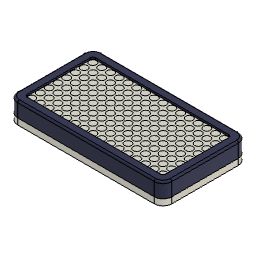
clock v5 (Autodesk Fusion 360 design; units mm, degrees)
Autodesk Fusion 360 part; units mm, degrees
(part 1 of 4)
sketch "Sketch1" plane through (0, 0, 0) normal (0, 0, 1) x (1, 0, 0)
  line L0 (1, 8.4943) -> (1, 1.4943)
  line L1 (1, 1.4943) -> (9, 1.4943)
  line L2 (9, 1.4943) -> (9, 8.4943)
  line L3 (9, 8.4943) -> (1, 8.4943)
  line L4 (19, 1.4943) -> (19, 8.4943)
  line L5 (19, 8.4943) -> (11, 8.4943)
  line L6 (11, 8.4943) -> (11, 1.4943)
  line L7 (11, 1.4943) -> (19, 1.4943)
  line L8 (29, 1.4943) -> (29, 8.4943)
  line L9 (29, 8.4943) -> (21, 8.4943)
  line L10 (21, 8.4943) -> (21, 1.4943)
  line L11 (21, 1.4943) -> (29, 1.4943)
  line L12 (39, 1.4943) -> (39, 8.4943)
  line L13 (39, 8.4943) -> (31, 8.4943)
  line L14 (31, 8.4943) -> (31, 1.4943)
  line L15 (31, 1.4943) -> (39, 1.4943)
  line L16 (49, 1.4943) -> (49, 8.4943)
  line L17 (49, 8.4943) -> (41, 8.4943)
  line L18 (41, 8.4943) -> (41, 1.4943)
  line L19 (41, 1.4943) -> (49, 1.4943)
  line L20 (59, 1.4943) -> (59, 8.4943)
  line L21 (59, 8.4943) -> (51, 8.4943)
  line L22 (51, 8.4943) -> (51, 1.4943)
  line L23 (51, 1.4943) -> (59, 1.4943)
  line L24 (69, 1.4943) -> (69, 8.4943)
  line L25 (69, 8.4943) -> (61, 8.4943)
  line L26 (61, 8.4943) -> (61, 1.4943)
  line L27 (61, 1.4943) -> (69, 1.4943)
  line L28 (79, 1.4943) -> (79, 8.4943)
  line L29 (79, 8.4943) -> (71, 8.4943)
  line L30 (71, 8.4943) -> (71, 1.4943)
  line L31 (71, 1.4943) -> (79, 1.4943)
  line L32 (89, 1.4943) -> (89, 8.4943)
  line L33 (89, 8.4943) -> (81, 8.4943)
  line L34 (81, 8.4943) -> (81, 1.4943)
  line L35 (81, 1.4943) -> (89, 1.4943)
  line L36 (99, 1.4943) -> (99, 8.4943)
  line L37 (99, 8.4943) -> (91, 8.4943)
  line L38 (91, 8.4943) -> (91, 1.4943)
  line L39 (91, 1.4943) -> (99, 1.4943)
  line L40 (109, 1.4943) -> (109, 8.4943)
  line L41 (109, 8.4943) -> (101, 8.4943)
  line L42 (101, 8.4943) -> (101, 1.4943)
  line L43 (101, 1.4943) -> (109, 1.4943)
  line L44 (119, 1.4943) -> (119, 8.4943)
  line L45 (119, 8.4943) -> (111, 8.4943)
  line L46 (111, 8.4943) -> (111, 1.4943)
  line L47 (111, 1.4943) -> (119, 1.4943)
  line L48 (129, 1.4943) -> (129, 8.4943)
  line L49 (129, 8.4943) -> (121, 8.4943)
  line L50 (121, 8.4943) -> (121, 1.4943)
  line L51 (121, 1.4943) -> (129, 1.4943)
  line L52 (139, 1.4943) -> (139, 8.4943)
  line L53 (139, 8.4943) -> (131, 8.4943)
  line L54 (131, 8.4943) -> (131, 1.4943)
  line L55 (131, 1.4943) -> (139, 1.4943)
  line L56 (149, 1.4943) -> (149, 8.4943)
  line L57 (149, 8.4943) -> (141, 8.4943)
  line L58 (141, 8.4943) -> (141, 1.4943)
  line L59 (141, 1.4943) -> (149, 1.4943)
  line L60 (159, 1.4943) -> (159, 8.4943)
  line L61 (159, 8.4943) -> (151, 8.4943)
  line L62 (151, 8.4943) -> (151, 1.4943)
  line L63 (151, 1.4943) -> (159, 1.4943)
  line L64 (9, 11.4943) -> (9, 18.4943)
  line L65 (9, 18.4943) -> (1, 18.4943)
  line L66 (1, 18.4943) -> (1, 11.4943)
  line L67 (1, 11.4943) -> (9, 11.4943)
  line L68 (19, 11.4943) -> (19, 18.4943)
  line L69 (19, 18.4943) -> (11, 18.4943)
  line L70 (11, 18.4943) -> (11, 11.4943)
  line L71 (11, 11.4943) -> (19, 11.4943)
  line L72 (29, 11.4943) -> (29, 18.4943)
  line L73 (29, 18.4943) -> (21, 18.4943)
  line L74 (21, 18.4943) -> (21, 11.4943)
  line L75 (21, 11.4943) -> (29, 11.4943)
  line L76 (39, 11.4943) -> (39, 18.4943)
  line L77 (39, 18.4943) -> (31, 18.4943)
  line L78 (31, 18.4943) -> (31, 11.4943)
  line L79 (31, 11.4943) -> (39, 11.4943)
  line L80 (49, 11.4943) -> (49, 18.4943)
  line L81 (49, 18.4943) -> (41, 18.4943)
  line L82 (41, 18.4943) -> (41, 11.4943)
  line L83 (41, 11.4943) -> (49, 11.4943)
  line L84 (59, 11.4943) -> (59, 18.4943)
  line L85 (59, 18.4943) -> (51, 18.4943)
  line L86 (51, 18.4943) -> (51, 11.4943)
  line L87 (51, 11.4943) -> (59, 11.4943)
  line L88 (69, 11.4943) -> (69, 18.4943)
  line L89 (69, 18.4943) -> (61, 18.4943)
  line L90 (61, 18.4943) -> (61, 11.4943)
  line L91 (61, 11.4943) -> (69, 11.4943)
  line L92 (79, 11.4943) -> (79, 18.4943)
  line L93 (79, 18.4943) -> (71, 18.4943)
  line L94 (71, 18.4943) -> (71, 11.4943)
  line L95 (71, 11.4943) -> (79, 11.4943)
  line L96 (89, 11.4943) -> (89, 18.4943)
  line L97 (89, 18.4943) -> (81, 18.4943)
  line L98 (81, 18.4943) -> (81, 11.4943)
  line L99 (81, 11.4943) -> (89, 11.4943)
  line L100 (99, 11.4943) -> (99, 18.4943)
  line L101 (99, 18.4943) -> (91, 18.4943)
  line L102 (91, 18.4943) -> (91, 11.4943)
  line L103 (91, 11.4943) -> (99, 11.4943)
  line L104 (109, 11.4943) -> (109, 18.4943)
  line L105 (109, 18.4943) -> (101, 18.4943)
  line L106 (101, 18.4943) -> (101, 11.4943)
  line L107 (101, 11.4943) -> (109, 11.4943)
  line L108 (119, 11.4943) -> (119, 18.4943)
  line L109 (119, 18.4943) -> (111, 18.4943)
  line L110 (111, 18.4943) -> (111, 11.4943)
  line L111 (111, 11.4943) -> (119, 11.4943)
  line L112 (129, 11.4943) -> (129, 18.4943)
  line L113 (129, 18.4943) -> (121, 18.4943)
  line L114 (121, 18.4943) -> (121, 11.4943)
  line L115 (121, 11.4943) -> (129, 11.4943)
  line L116 (139, 11.4943) -> (139, 18.4943)
  line L117 (139, 18.4943) -> (131, 18.4943)
  line L118 (131, 18.4943) -> (131, 11.4943)
  line L119 (131, 11.4943) -> (139, 11.4943)
  line L120 (149, 11.4943) -> (149, 18.4943)
  line L121 (149, 18.4943) -> (141, 18.4943)
  line L122 (141, 18.4943) -> (141, 11.4943)
  line L123 (141, 11.4943) -> (149, 11.4943)
  line L124 (159, 11.4943) -> (159, 18.4943)
  line L125 (159, 18.4943) -> (151, 18.4943)
  line L126 (151, 18.4943) -> (151, 11.4943)
  line L127 (151, 11.4943) -> (159, 11.4943)
  line L128 (9, 21.4943) -> (9, 28.4943)
  line L129 (9, 28.4943) -> (1, 28.4943)
  line L130 (1, 28.4943) -> (1, 21.4943)
  line L131 (1, 21.4943) -> (9, 21.4943)
  line L132 (19, 21.4943) -> (19, 28.4943)
  line L133 (19, 28.4943) -> (11, 28.4943)
  line L134 (11, 28.4943) -> (11, 21.4943)
  line L135 (11, 21.4943) -> (19, 21.4943)
  line L136 (29, 21.4943) -> (29, 28.4943)
  line L137 (29, 28.4943) -> (21, 28.4943)
  line L138 (21, 28.4943) -> (21, 21.4943)
  line L139 (21, 21.4943) -> (29, 21.4943)
  line L140 (39, 21.4943) -> (39, 28.4943)
  line L141 (39, 28.4943) -> (31, 28.4943)
  line L142 (31, 28.4943) -> (31, 21.4943)
  line L143 (31, 21.4943) -> (39, 21.4943)
  line L144 (49, 21.4943) -> (49, 28.4943)
  line L145 (49, 28.4943) -> (41, 28.4943)
  line L146 (41, 28.4943) -> (41, 21.4943)
  line L147 (41, 21.4943) -> (49, 21.4943)
  line L148 (59, 21.4943) -> (59, 28.4943)
  line L149 (59, 28.4943) -> (51, 28.4943)
  line L150 (51, 28.4943) -> (51, 21.4943)
  line L151 (51, 21.4943) -> (59, 21.4943)
  line L152 (69, 21.4943) -> (69, 28.4943)
  line L153 (69, 28.4943) -> (61, 28.4943)
  line L154 (61, 28.4943) -> (61, 21.4943)
  line L155 (61, 21.4943) -> (69, 21.4943)
  line L156 (79, 21.4943) -> (79, 28.4943)
  line L157 (79, 28.4943) -> (71, 28.4943)
  line L158 (71, 28.4943) -> (71, 21.4943)
  line L159 (71, 21.4943) -> (79, 21.4943)
  line L160 (89, 21.4943) -> (89, 28.4943)
  line L161 (89, 28.4943) -> (81, 28.4943)
  line L162 (81, 28.4943) -> (81, 21.4943)
  line L163 (81, 21.4943) -> (89, 21.4943)
  line L164 (99, 21.4943) -> (99, 28.4943)
  line L165 (99, 28.4943) -> (91, 28.4943)
  line L166 (91, 28.4943) -> (91, 21.4943)
  line L167 (91, 21.4943) -> (99, 21.4943)
  line L168 (109, 21.4943) -> (109, 28.4943)
  line L169 (109, 28.4943) -> (101, 28.4943)
  line L170 (101, 28.4943) -> (101, 21.4943)
  line L171 (101, 21.4943) -> (109, 21.4943)
  line L172 (119, 21.4943) -> (119, 28.4943)
  line L173 (119, 28.4943) -> (111, 28.4943)
  line L174 (111, 28.4943) -> (111, 21.4943)
  line L175 (111, 21.4943) -> (119, 21.4943)
  line L176 (129, 21.4943) -> (129, 28.4943)
  line L177 (129, 28.4943) -> (121, 28.4943)
  line L178 (121, 28.4943) -> (121, 21.4943)
  line L179 (121, 21.4943) -> (129, 21.4943)
  line L180 (139, 21.4943) -> (139, 28.4943)
  line L181 (139, 28.4943) -> (131, 28.4943)
  line L182 (131, 28.4943) -> (131, 21.4943)
  line L183 (131, 21.4943) -> (139, 21.4943)
  line L184 (149, 21.4943) -> (149, 28.4943)
  line L185 (149, 28.4943) -> (141, 28.4943)
  line L186 (141, 28.4943) -> (141, 21.4943)
  line L187 (141, 21.4943) -> (149, 21.4943)
  line L188 (159, 21.4943) -> (159, 28.4943)
  line L189 (159, 28.4943) -> (151, 28.4943)
  line L190 (151, 28.4943) -> (151, 21.4943)
  line L191 (151, 21.4943) -> (159, 21.4943)
  line L192 (9, 31.4943) -> (9, 38.4943)
  line L193 (9, 38.4943) -> (1, 38.4943)
  line L194 (1, 38.4943) -> (1, 31.4943)
  line L195 (1, 31.4943) -> (9, 31.4943)
  line L196 (19, 31.4943) -> (19, 38.4943)
  line L197 (19, 38.4943) -> (11, 38.4943)
  line L198 (11, 38.4943) -> (11, 31.4943)
  line L199 (11, 31.4943) -> (19, 31.4943)
  line L200 (29, 31.4943) -> (29, 38.4943)
  line L201 (29, 38.4943) -> (21, 38.4943)
  line L202 (21, 38.4943) -> (21, 31.4943)
  line L203 (21, 31.4943) -> (29, 31.4943)
  line L204 (39, 31.4943) -> (39, 38.4943)
  line L205 (39, 38.4943) -> (31, 38.4943)
  line L206 (31, 38.4943) -> (31, 31.4943)
  line L207 (31, 31.4943) -> (39, 31.4943)
  line L208 (49, 31.4943) -> (49, 38.4943)
  line L209 (49, 38.4943) -> (41, 38.4943)
  line L210 (41, 38.4943) -> (41, 31.4943)
  line L211 (41, 31.4943) -> (49, 31.4943)
  line L212 (59, 31.4943) -> (59, 38.4943)
  line L213 (59, 38.4943) -> (51, 38.4943)
  line L214 (51, 38.4943) -> (51, 31.4943)
  line L215 (51, 31.4943) -> (59, 31.4943)
  line L216 (69, 31.4943) -> (69, 38.4943)
  line L217 (69, 38.4943) -> (61, 38.4943)
  line L218 (61, 38.4943) -> (61, 31.4943)
  line L219 (61, 31.4943) -> (69, 31.4943)
  line L220 (79, 31.4943) -> (79, 38.4943)
  line L221 (79, 38.4943) -> (71, 38.4943)
  line L222 (71, 38.4943) -> (71, 31.4943)
  line L223 (71, 31.4943) -> (79, 31.4943)
  line L224 (89, 31.4943) -> (89, 38.4943)
  line L225 (89, 38.4943) -> (81, 38.4943)
  line L226 (81, 38.4943) -> (81, 31.4943)
  line L227 (81, 31.4943) -> (89, 31.4943)
  line L228 (99, 31.4943) -> (99, 38.4943)
  line L229 (99, 38.4943) -> (91, 38.4943)
  line L230 (91, 38.4943) -> (91, 31.4943)
  line L231 (91, 31.4943) -> (99, 31.4943)
  line L232 (109, 31.4943) -> (109, 38.4943)
  line L233 (109, 38.4943) -> (101, 38.4943)
  line L234 (101, 38.4943) -> (101, 31.4943)
  line L235 (101, 31.4943) -> (109, 31.4943)
  line L236 (119, 31.4943) -> (119, 38.4943)
  line L237 (119, 38.4943) -> (111, 38.4943)
  line L238 (111, 38.4943) -> (111, 31.4943)
  line L239 (111, 31.4943) -> (119, 31.4943)
  line L240 (129, 31.4943) -> (129, 38.4943)
  line L241 (129, 38.4943) -> (121, 38.4943)
  line L242 (121, 38.4943) -> (121, 31.4943)
  line L243 (121, 31.4943) -> (129, 31.4943)
  line L244 (139, 31.4943) -> (139, 38.4943)
  line L245 (139, 38.4943) -> (131, 38.4943)
  line L246 (131, 38.4943) -> (131, 31.4943)
  line L247 (131, 31.4943) -> (139, 31.4943)
  line L248 (149, 31.4943) -> (149, 38.4943)
  line L249 (149, 38.4943) -> (141, 38.4943)
  line L250 (141, 38.4943) -> (141, 31.4943)
  line L251 (141, 31.4943) -> (149, 31.4943)
  line L252 (159, 31.4943) -> (159, 38.4943)
  line L253 (159, 38.4943) -> (151, 38.4943)
  line L254 (151, 38.4943) -> (151, 31.4943)
  line L255 (151, 31.4943) -> (159, 31.4943)
  line L256 (9, 41.4943) -> (9, 48.4943)
  line L257 (9, 48.4943) -> (1, 48.4943)
  line L258 (1, 48.4943) -> (1, 41.4943)
  line L259 (1, 41.4943) -> (9, 41.4943)
  line L260 (19, 41.4943) -> (19, 48.4943)
  line L261 (19, 48.4943) -> (11, 48.4943)
  line L262 (11, 48.4943) -> (11, 41.4943)
  line L263 (11, 41.4943) -> (19, 41.4943)
  line L264 (29, 41.4943) -> (29, 48.4943)
  line L265 (29, 48.4943) -> (21, 48.4943)
  line L266 (21, 48.4943) -> (21, 41.4943)
  line L267 (21, 41.4943) -> (29, 41.4943)
  line L268 (39, 41.4943) -> (39, 48.4943)
  line L269 (39, 48.4943) -> (31, 48.4943)
  line L270 (31, 48.4943) -> (31, 41.4943)
  line L271 (31, 41.4943) -> (39, 41.4943)
  line L272 (49, 41.4943) -> (49, 48.4943)
  line L273 (49, 48.4943) -> (41, 48.4943)
  line L274 (41, 48.4943) -> (41, 41.4943)
  line L275 (41, 41.4943) -> (49, 41.4943)
  line L276 (59, 41.4943) -> (59, 48.4943)
  line L277 (59, 48.4943) -> (51, 48.4943)
  line L278 (51, 48.4943) -> (51, 41.4943)
  line L279 (51, 41.4943) -> (59, 41.4943)
  line L280 (69, 41.4943) -> (69, 48.4943)
  line L281 (69, 48.4943) -> (61, 48.4943)
  line L282 (61, 48.4943) -> (61, 41.4943)
  line L283 (61, 41.4943) -> (69, 41.4943)
  line L284 (79, 41.4943) -> (79, 48.4943)
  line L285 (79, 48.4943) -> (71, 48.4943)
  line L286 (71, 48.4943) -> (71, 41.4943)
  line L287 (71, 41.4943) -> (79, 41.4943)
  line L288 (89, 41.4943) -> (89, 48.4943)
  line L289 (89, 48.4943) -> (81, 48.4943)
  line L290 (81, 48.4943) -> (81, 41.4943)
  line L291 (81, 41.4943) -> (89, 41.4943)
  line L292 (99, 41.4943) -> (99, 48.4943)
  line L293 (99, 48.4943) -> (91, 48.4943)
  line L294 (91, 48.4943) -> (91, 41.4943)
  line L295 (91, 41.4943) -> (99, 41.4943)
  line L296 (109, 41.4943) -> (109, 48.4943)
  line L297 (109, 48.4943) -> (101, 48.4943)
  line L298 (101, 48.4943) -> (101, 41.4943)
  line L299 (101, 41.4943) -> (109, 41.4943)
  line L300 (119, 41.4943) -> (119, 48.4943)
  line L301 (119, 48.4943) -> (111, 48.4943)
  line L302 (111, 48.4943) -> (111, 41.4943)
  line L303 (111, 41.4943) -> (119, 41.4943)
  line L304 (129, 41.4943) -> (129, 48.4943)
  line L305 (129, 48.4943) -> (121, 48.4943)
  line L306 (121, 48.4943) -> (121, 41.4943)
  line L307 (121, 41.4943) -> (129, 41.4943)
  line L308 (139, 41.4943) -> (139, 48.4943)
  line L309 (139, 48.4943) -> (131, 48.4943)
  line L310 (131, 48.4943) -> (131, 41.4943)
  line L311 (131, 41.4943) -> (139, 41.4943)
  line L312 (149, 41.4943) -> (149, 48.4943)
  line L313 (149, 48.4943) -> (141, 48.4943)
  line L314 (141, 48.4943) -> (141, 41.4943)
  line L315 (141, 41.4943) -> (149, 41.4943)
  line L316 (159, 41.4943) -> (159, 48.4943)
  line L317 (159, 48.4943) -> (151, 48.4943)
  line L318 (151, 48.4943) -> (151, 41.4943)
  line L319 (151, 41.4943) -> (159, 41.4943)
  line L320 (9, 51.4943) -> (9, 58.4943)
  line L321 (9, 58.4943) -> (1, 58.4943)
  line L322 (1, 58.4943) -> (1, 51.4943)
  line L323 (1, 51.4943) -> (9, 51.4943)
  line L324 (19, 51.4943) -> (19, 58.4943)
  line L325 (19, 58.4943) -> (11, 58.4943)
  line L326 (11, 58.4943) -> (11, 51.4943)
  line L327 (11, 51.4943) -> (19, 51.4943)
  line L328 (29, 51.4943) -> (29, 58.4943)
  line L329 (29, 58.4943) -> (21, 58.4943)
  line L330 (21, 58.4943) -> (21, 51.4943)
  line L331 (21, 51.4943) -> (29, 51.4943)
  line L332 (39, 51.4943) -> (39, 58.4943)
  line L333 (39, 58.4943) -> (31, 58.4943)
  line L334 (31, 58.4943) -> (31, 51.4943)
  line L335 (31, 51.4943) -> (39, 51.4943)
  line L336 (49, 51.4943) -> (49, 58.4943)
  line L337 (49, 58.4943) -> (41, 58.4943)
  line L338 (41, 58.4943) -> (41, 51.4943)
  line L339 (41, 51.4943) -> (49, 51.4943)
  line L340 (59, 51.4943) -> (59, 58.4943)
  line L341 (59, 58.4943) -> (51, 58.4943)
  line L342 (51, 58.4943) -> (51, 51.4943)
  line L343 (51, 51.4943) -> (59, 51.4943)
  line L344 (69, 51.4943) -> (69, 58.4943)
  line L345 (69, 58.4943) -> (61, 58.4943)
  line L346 (61, 58.4943) -> (61, 51.4943)
  line L347 (61, 51.4943) -> (69, 51.4943)
  line L348 (79, 51.4943) -> (79, 58.4943)
  line L349 (79, 58.4943) -> (71, 58.4943)
  line L350 (71, 58.4943) -> (71, 51.4943)
  line L351 (71, 51.4943) -> (79, 51.4943)
  line L352 (89, 51.4943) -> (89, 58.4943)
  line L353 (89, 58.4943) -> (81, 58.4943)
  line L354 (81, 58.4943) -> (81, 51.4943)
  line L355 (81, 51.4943) -> (89, 51.4943)
  line L356 (99, 51.4943) -> (99, 58.4943)
  line L357 (99, 58.4943) -> (91, 58.4943)
  line L358 (91, 58.4943) -> (91, 51.4943)
  line L359 (91, 51.4943) -> (99, 51.4943)
  line L360 (109, 51.4943) -> (109, 58.4943)
  line L361 (109, 58.4943) -> (101, 58.4943)
  line L362 (101, 58.4943) -> (101, 51.4943)
  line L363 (101, 51.4943) -> (109, 51.4943)
  line L364 (119, 51.4943) -> (119, 58.4943)
  line L365 (119, 58.4943) -> (111, 58.4943)
  line L366 (111, 58.4943) -> (111, 51.4943)
  line L367 (111, 51.4943) -> (119, 51.4943)
  line L368 (129, 51.4943) -> (129, 58.4943)
  line L369 (129, 58.4943) -> (121, 58.4943)
  line L370 (121, 58.4943) -> (121, 51.4943)
  line L371 (121, 51.4943) -> (129, 51.4943)
  line L372 (139, 51.4943) -> (139, 58.4943)
  line L373 (139, 58.4943) -> (131, 58.4943)
  line L374 (131, 58.4943) -> (131, 51.4943)
  line L375 (131, 51.4943) -> (139, 51.4943)
  line L376 (149, 51.4943) -> (149, 58.4943)
  line L377 (149, 58.4943) -> (141, 58.4943)
  line L378 (141, 58.4943) -> (141, 51.4943)
  line L379 (141, 51.4943) -> (149, 51.4943)
  line L380 (159, 51.4943) -> (159, 58.4943)
  line L381 (159, 58.4943) -> (151, 58.4943)
  line L382 (151, 58.4943) -> (151, 51.4943)
  line L383 (151, 51.4943) -> (159, 51.4943)
  line L384 (9, 61.4943) -> (9, 68.4943)
  line L385 (9, 68.4943) -> (1, 68.4943)
  line L386 (1, 68.4943) -> (1, 61.4943)
  line L387 (1, 61.4943) -> (9, 61.4943)
  line L388 (19, 61.4943) -> (19, 68.4943)
  line L389 (19, 68.4943) -> (11, 68.4943)
  line L390 (11, 68.4943) -> (11, 61.4943)
  line L391 (11, 61.4943) -> (19, 61.4943)
  line L392 (29, 61.4943) -> (29, 68.4943)
  line L393 (29, 68.4943) -> (21, 68.4943)
  line L394 (21, 68.4943) -> (21, 61.4943)
  line L395 (21, 61.4943) -> (29, 61.4943)
  line L396 (39, 61.4943) -> (39, 68.4943)
  line L397 (39, 68.4943) -> (31, 68.4943)
  line L398 (31, 68.4943) -> (31, 61.4943)
  line L399 (31, 61.4943) -> (39, 61.4943)
  line L400 (49, 61.4943) -> (49, 68.4943)
  line L401 (49, 68.4943) -> (41, 68.4943)
  line L402 (41, 68.4943) -> (41, 61.4943)
  line L403 (41, 61.4943) -> (49, 61.4943)
  line L404 (59, 61.4943) -> (59, 68.4943)
  line L405 (59, 68.4943) -> (51, 68.4943)
  line L406 (51, 68.4943) -> (51, 61.4943)
  line L407 (51, 61.4943) -> (59, 61.4943)
  line L408 (69, 61.4943) -> (69, 68.4943)
  line L409 (69, 68.4943) -> (61, 68.4943)
  line L410 (61, 68.4943) -> (61, 61.4943)
  line L411 (61, 61.4943) -> (69, 61.4943)
  line L412 (79, 61.4943) -> (79, 68.4943)
  line L413 (79, 68.4943) -> (71, 68.4943)
  line L414 (71, 68.4943) -> (71, 61.4943)
  line L415 (71, 61.4943) -> (79, 61.4943)
  line L416 (89, 61.4943) -> (89, 68.4943)
  line L417 (89, 68.4943) -> (81, 68.4943)
  line L418 (81, 68.4943) -> (81, 61.4943)
  line L419 (81, 61.4943) -> (89, 61.4943)
  line L420 (99, 61.4943) -> (99, 68.4943)
  line L421 (99, 68.4943) -> (91, 68.4943)
  line L422 (91, 68.4943) -> (91, 61.4943)
  line L423 (91, 61.4943) -> (99, 61.4943)
  line L424 (109, 61.4943) -> (109, 68.4943)
  line L425 (109, 68.4943) -> (101, 68.4943)
  line L426 (101, 68.4943) -> (101, 61.4943)
  line L427 (101, 61.4943) -> (109, 61.4943)
  line L428 (119, 61.4943) -> (119, 68.4943)
  line L429 (119, 68.4943) -> (111, 68.4943)
  line L430 (111, 68.4943) -> (111, 61.4943)
  line L431 (111, 61.4943) -> (119, 61.4943)
  line L432 (129, 61.4943) -> (129, 68.4943)
  line L433 (129, 68.4943) -> (121, 68.4943)
  line L434 (121, 68.4943) -> (121, 61.4943)
  line L435 (121, 61.4943) -> (129, 61.4943)
  line L436 (139, 61.4943) -> (139, 68.4943)
  line L437 (139, 68.4943) -> (131, 68.4943)
  line L438 (131, 68.4943) -> (131, 61.4943)
  line L439 (131, 61.4943) -> (139, 61.4943)
  line L440 (149, 61.4943) -> (149, 68.4943)
  line L441 (149, 68.4943) -> (141, 68.4943)
  line L442 (141, 68.4943) -> (141, 61.4943)
  line L443 (141, 61.4943) -> (149, 61.4943)
  line L444 (159, 61.4943) -> (159, 68.4943)
  line L445 (159, 68.4943) -> (151, 68.4943)
  line L446 (151, 68.4943) -> (151, 61.4943)
  line L447 (151, 61.4943) -> (159, 61.4943)
  line L448 (9, 71.4943) -> (9, 78.4943)
  line L449 (9, 78.4943) -> (1, 78.4943)
  line L450 (1, 78.4943) -> (1, 71.4943)
  line L451 (1, 71.4943) -> (9, 71.4943)
  line L452 (19, 71.4943) -> (19, 78.4943)
  line L453 (19, 78.4943) -> (11, 78.4943)
  line L454 (11, 78.4943) -> (11, 71.4943)
  line L455 (11, 71.4943) -> (19, 71.4943)
  line L456 (29, 71.4943) -> (29, 78.4943)
  line L457 (29, 78.4943) -> (21, 78.4943)
  line L458 (21, 78.4943) -> (21, 71.4943)
  line L459 (21, 71.4943) -> (29, 71.4943)
  line L460 (39, 71.4943) -> (39, 78.4943)
  line L461 (39, 78.4943) -> (31, 78.4943)
  line L462 (31, 78.4943) -> (31, 71.4943)
  line L463 (31, 71.4943) -> (39, 71.4943)
  line L464 (49, 71.4943) -> (49, 78.4943)
  line L465 (49, 78.4943) -> (41, 78.4943)
  line L466 (41, 78.4943) -> (41, 71.4943)
  line L467 (41, 71.4943) -> (49, 71.4943)
  line L468 (59, 71.4943) -> (59, 78.4943)
  line L469 (59, 78.4943) -> (51, 78.4943)
  line L470 (51, 78.4943) -> (51, 71.4943)
  line L471 (51, 71.4943) -> (59, 71.4943)
  line L472 (69, 71.4943) -> (69, 78.4943)
  line L473 (69, 78.4943) -> (61, 78.4943)
  line L474 (61, 78.4943) -> (61, 71.4943)
  line L475 (61, 71.4943) -> (69, 71.4943)
  line L476 (79, 71.4943) -> (79, 78.4943)
  line L477 (79, 78.4943) -> (71, 78.4943)
  line L478 (71, 78.4943) -> (71, 71.4943)
  line L479 (71, 71.4943) -> (79, 71.4943)
  line L480 (89, 71.4943) -> (89, 78.4943)
  line L481 (89, 78.4943) -> (81, 78.4943)
  line L482 (81, 78.4943) -> (81, 71.4943)
  line L483 (81, 71.4943) -> (89, 71.4943)
  line L484 (99, 71.4943) -> (99, 78.4943)
  line L485 (99, 78.4943) -> (91, 78.4943)
  line L486 (91, 78.4943) -> (91, 71.4943)
  line L487 (91, 71.4943) -> (99, 71.4943)
  line L488 (109, 71.4943) -> (109, 78.4943)
  line L489 (109, 78.4943) -> (101, 78.4943)
  line L490 (101, 78.4943) -> (101, 71.4943)
  line L491 (101, 71.4943) -> (109, 71.4943)
  line L492 (119, 71.4943) -> (119, 78.4943)
  line L493 (119, 78.4943) -> (111, 78.4943)
  line L494 (111, 78.4943) -> (111, 71.4943)
  line L495 (111, 71.4943) -> (119, 71.4943)
  line L496 (129, 71.4943) -> (129, 78.4943)
  line L497 (129, 78.4943) -> (121, 78.4943)
  line L498 (121, 78.4943) -> (121, 71.4943)
  line L499 (121, 71.4943) -> (129, 71.4943)
  line L500 (139, 71.4943) -> (139, 78.4943)
  line L501 (139, 78.4943) -> (131, 78.4943)
  line L502 (131, 78.4943) -> (131, 71.4943)
  line L503 (131, 71.4943) -> (139, 71.4943)
  line L504 (149, 71.4943) -> (149, 78.4943)
  line L505 (149, 78.4943) -> (141, 78.4943)
  line L506 (141, 78.4943) -> (141, 71.4943)
  line L507 (141, 71.4943) -> (149, 71.4943)
  line L508 (159, 71.4943) -> (159, 78.4943)
  line L509 (159, 78.4943) -> (151, 78.4943)
  line L510 (151, 78.4943) -> (151, 71.4943)
  line L511 (151, 71.4943) -> (159, 71.4943)
  line L512 (161, -1) -> (161, 81)
  line L513 (161, 81) -> (-1, 81)
  line L514 (-1, 81) -> (-1, -1)
  line L515 (-1, -1) -> (161, -1)
  dimension "d6" = 150
  dimension "d7" = 70
  dimension "d39" = 7
  measures "d39" distance of L0.start L0.end
ref_plane "WorkPlane1" through (80, 40, 10) normal (0, 0, 1) x (1, 0, 0)
sketch "Sketch2" plane through (80, 40, 10) normal (0, 0, 1) x (1, 0, 0)
  circle A0 centre (-75, -35) radius 4
  line L0 (-81, -41) -> (81, -41)
  line L1 (81, -41) -> (81, 41)
  line L2 (81, 41) -> (-81, 41)
  line L3 (-81, 41) -> (-81, -41)
  circle A1 centre (-65, -35) radius 4
  circle A2 centre (-55, -35) radius 4
  circle A3 centre (-45, -35) radius 4
  circle A4 centre (-35, -35) radius 4
  circle A5 centre (-25, -35) radius 4
  circle A6 centre (-15, -35) radius 4
  circle A7 centre (-5, -35) radius 4
  circle A8 centre (5, -35) radius 4
  circle A9 centre (15, -35) radius 4
  circle A10 centre (25, -35) radius 4
  circle A11 centre (35, -35) radius 4
  circle A12 centre (45, -35) radius 4
  circle A13 centre (55, -35) radius 4
  circle A14 centre (65, -35) radius 4
  circle A15 centre (75, -35) radius 4
  circle A16 centre (-75, -25) radius 4
  circle A17 centre (-65, -25) radius 4
  circle A18 centre (-55, -25) radius 4
  circle A19 centre (-45, -25) radius 4
  circle A20 centre (-35, -25) radius 4
  circle A21 centre (-25, -25) radius 4
  circle A22 centre (-15, -25) radius 4
  circle A23 centre (-5, -25) radius 4
  circle A24 centre (5, -25) radius 4
  circle A25 centre (15, -25) radius 4
  circle A26 centre (25, -25) radius 4
  circle A27 centre (35, -25) radius 4
  circle A28 centre (45, -25) radius 4
  circle A29 centre (55, -25) radius 4
  circle A30 centre (65, -25) radius 4
  circle A31 centre (75, -25) radius 4
  circle A32 centre (-75, -15) radius 4
  circle A33 centre (-65, -15) radius 4
  circle A34 centre (-55, -15) radius 4
  circle A35 centre (-45, -15) radius 4
  circle A36 centre (-35, -15) radius 4
  circle A37 centre (-25, -15) radius 4
  circle A38 centre (-15, -15) radius 4
  circle A39 centre (-5, -15) radius 4
  circle A40 centre (5, -15) radius 4
  circle A41 centre (15, -15) radius 4
  circle A42 centre (25, -15) radius 4
  circle A43 centre (35, -15) radius 4
  circle A44 centre (45, -15) radius 4
  circle A45 centre (55, -15) radius 4
  circle A46 centre (65, -15) radius 4
  circle A47 centre (75, -15) radius 4
  circle A48 centre (-75, -5) radius 4
  circle A49 centre (-65, -5) radius 4
  circle A50 centre (-55, -5) radius 4
  circle A51 centre (-45, -5) radius 4
  circle A52 centre (-35, -5) radius 4
  circle A53 centre (-25, -5) radius 4
  circle A54 centre (-15, -5) radius 4
  circle A55 centre (-5, -5) radius 4
  circle A56 centre (5, -5) radius 4
  circle A57 centre (15, -5) radius 4
  circle A58 centre (25, -5) radius 4
  circle A59 centre (35, -5) radius 4
  circle A60 centre (45, -5) radius 4
  circle A61 centre (55, -5) radius 4
  circle A62 centre (65, -5) radius 4
  circle A63 centre (75, -5) radius 4
  circle A64 centre (-75, 5) radius 4
  circle A65 centre (-65, 5) radius 4
  circle A66 centre (-55, 5) radius 4
  circle A67 centre (-45, 5) radius 4
  circle A68 centre (-35, 5) radius 4
  circle A69 centre (-25, 5) radius 4
  circle A70 centre (-15, 5) radius 4
  circle A71 centre (-5, 5) radius 4
  circle A72 centre (5, 5) radius 4
  circle A73 centre (15, 5) radius 4
  circle A74 centre (25, 5) radius 4
  circle A75 centre (35, 5) radius 4
  circle A76 centre (45, 5) radius 4
  circle A77 centre (55, 5) radius 4
  circle A78 centre (65, 5) radius 4
  circle A79 centre (75, 5) radius 4
  circle A80 centre (-75, 15) radius 4
  circle A81 centre (-65, 15) radius 4
  circle A82 centre (-55, 15) radius 4
  circle A83 centre (-45, 15) radius 4
  circle A84 centre (-35, 15) radius 4
  circle A85 centre (-25, 15) radius 4
  circle A86 centre (-15, 15) radius 4
  circle A87 centre (-5, 15) radius 4
  circle A88 centre (5, 15) radius 4
  circle A89 centre (15, 15) radius 4
  circle A90 centre (25, 15) radius 4
  circle A91 centre (35, 15) radius 4
  circle A92 centre (45, 15) radius 4
  circle A93 centre (55, 15) radius 4
  circle A94 centre (65, 15) radius 4
  circle A95 centre (75, 15) radius 4
  circle A96 centre (-75, 25) radius 4
  circle A97 centre (-65, 25) radius 4
  circle A98 centre (-55, 25) radius 4
  circle A99 centre (-45, 25) radius 4
  circle A100 centre (-35, 25) radius 4
  circle A101 centre (-25, 25) radius 4
  circle A102 centre (-15, 25) radius 4
  circle A103 centre (-5, 25) radius 4
  circle A104 centre (5, 25) radius 4
  circle A105 centre (15, 25) radius 4
  circle A106 centre (25, 25) radius 4
  circle A107 centre (35, 25) radius 4
  circle A108 centre (45, 25) radius 4
  circle A109 centre (55, 25) radius 4
  circle A110 centre (65, 25) radius 4
  circle A111 centre (75, 25) radius 4
  circle A112 centre (-75, 35) radius 4
  circle A113 centre (-65, 35) radius 4
  circle A114 centre (-55, 35) radius 4
  circle A115 centre (-45, 35) radius 4
  circle A116 centre (-35, 35) radius 4
  circle A117 centre (-25, 35) radius 4
  circle A118 centre (-15, 35) radius 4
  circle A119 centre (-5, 35) radius 4
  circle A120 centre (5, 35) radius 4
  circle A121 centre (15, 35) radius 4
  circle A122 centre (25, 35) radius 4
  circle A123 centre (35, 35) radius 4
  circle A124 centre (45, 35) radius 4
  circle A125 centre (55, 35) radius 4
  circle A126 centre (65, 35) radius 4
  circle A127 centre (75, 35) radius 4
  dimension "d10" = 162
  dimension "d11" = 82
  dimension "d14" = 150
  dimension "d15" = 70
  constraint horizontal L0
  constraint vertical L1
  constraint horizontal L2
  constraint vertical L3
  measures "d10" distance of L0.start L0.end
  measures "d11" distance of L0.start L2.end
extrude "Extrude1" add sketch "Sketch1" along normal blind 10 contours L0 L1 L2 L3 | L4 L5 L6 L7 | L8 L9 L10 L11 | L12 L13 L14 L15 | L16 L17 L18 L19 | L20 L21 L22 L23 | L24 L25 L26 L27 | L28 L29 L30 L31 | L32 L33 L34 L35 | L36 L37 L38 L39 | L40 L41 L42 L43 | L44 L45 L46 L47 | L48 L49 L50 L51 | L52 L53 L54 L55 | L56 L57 L58 L59 | L60 L61 L62 L63 | L64 L65 L66 L67 | L68 L69 L70 L71 | L72 L73 L74 L75 | L76 L77 L78 L79 | L80 L81 L82 L83 | L84 L85 L86 L87 | L88 L89 L90 L91 | L92 L93 L94 L95 | L96 L97 L98 L99 | L100 L101 L102 L103 | L104 L105 L106 L107 | L108 L109 L110 L111 | L112 L113 L114 L115 | L116 L117 L118 L119 | L120 L121 L122 L123 | L124 L125 L126 L127 | L128 L129 L130 L131 | L132 L133 L134 L135 | L136 L137 L138 L139 | L140 L141 L142 L143 | L144 L145 L146 L147 | L148 L149 L150 L151 | L152 L153 L154 L155 | L156 L157 L158 L159 | L160 L161 L162 L163 | L164 L165 L166 L167 | L168 L169 L170 L171 | L172 L173 L174 L175 | L176 L177 L178 L179 | L180 L181 L182 L183 | L184 L185 L186 L187 | L188 L189 L190 L191 | L192 L193 L194 L195 | L196 L197 L198 L199 | L200 L201 L202 L203 | L204 L205 L206 L207 | L208 L209 L210 L211 | L212 L213 L214 L215 | L216 L217 L218 L219 | L220 L221 L222 L223 | L224 L225 L226 L227 | L228 L229 L230 L231 | L232 L233 L234 L235 | L236 L237 L238 L239 | L240 L241 L242 L243 | L244 L245 L246 L247 | L248 L249 L250 L251 | L252 L253 L254 L255 | L256 L257 L258 L259 | L260 L261 L262 L263 | L264 L265 L266 L267 | L268 L269 L270 L271 | L272 L273 L274 L275 | L276 L277 L278 L279 | L280 L281 L282 L283 | L284 L285 L286 L287 | L288 L289 L290 L291 | L292 L293 L294 L295 | L296 L297 L298 L299 | L300 L301 L302 L303 | L304 L305 L306 L307 | L308 L309 L310 L311 | L312 L313 L314 L315 | L316 L317 L318 L319 | L320 L321 L322 L323 | L324 L325 L326 L327 | L328 L329 L330 L331 | L332 L333 L334 L335 | L336 L337 L338 L339 | L340 L341 L342 L343 | L344 L345 L346 L347 | L348 L349 L350 L351 | L352 L353 L354 L355 | L356 L357 L358 L359 | L360 L361 L362 L363 | L364 L365 L366 L367 | L368 L369 L370 L371 | L372 L373 L374 L375 | L376 L377 L378 L379 | L380 L381 L382 L383 | L384 L385 L386 L387 | L388 L389 L390 L391 | L392 L393 L394 L395 | L396 L397 L398 L399 | L400 L401 L402 L403 | L404 L405 L406 L407 | L408 L409 L410 L411 | L412 L413 L414 L415 | L416 L417 L418 L419 | L420 L421 L422 L423 | L424 L425 L426 L427 | L428 L429 L430 L431 | L432 L433 L434 L435 | L436 L437 L438 L439 | L440 L441 L442 L443 | L444 L445 L446 L447 | L448 L449 L450 L451 | L452 L453 L454 L455 | L456 L457 L458 L459 | L460 L461 L462 L463 | L464 L465 L466 L467 | L468 L469 L470 L471 | L472 L473 L474 L475 | L476 L477 L478 L479 | L480 L481 L482 L483 | L484 L485 L486 L487 | L488 L489 L490 L491 | L492 L493 L494 L495 | L496 L497 L498 L499 | L500 L501 L502 L503 | L504 L505 L506 L507 | L508 L509 L510 L511 | L512 L513 L514 L515 makes body 1
loft "Loft1" cut profiles "Sketch1", "Sketch2" section 1 contours L0 L1 L2 L3 section 2 contours A0 bodies 1
pattern_linear "R-Pattern1" count 8 spacing 10 along (0, 1, 0) count 16 spacing 10 along (1, 0, 0) of "Loft1"
sketch "Sketch3" plane through (0, 0, 10) normal (0, 0, 1) x (-1, 0, 0)
  spline S0 degree 3 poles (-151.9897, -77.634) (-152.7286, -78.4785) (-153.8364, -78.9881) (-154.9584, -78.9998) (-156.1081, -79.0117) (-157.2531, -78.4994) (-158.0103, -77.634) knots -1 -1 -1 -1 -0.506107 -0.506107 -0.506107 0 0 0 0
  spline S1 degree 3 poles (-158.0103, -77.634) (-158.6337, -76.9215) (-158.9915, -75.9818) (-158.9998, -75.0351) (-159.0084, -74.065) (-158.6492, -73.0961) (-158.0103, -72.366) knots -1 -1 -1 -1 -0.506107 -0.506107 -0.506107 0 0 0 0
  spline S2 degree 3 poles (-158.0103, -72.366) (-157.2714, -71.5215) (-156.1636, -71.0119) (-155.0416, -71.0002) (-153.8919, -70.9883) (-152.7469, -71.5006) (-151.9897, -72.366) knots -1 -1 -1 -1 -0.506107 -0.506107 -0.506107 0 0 0 0
  spline S3 degree 3 poles (-151.9897, -72.366) (-151.3663, -73.0785) (-151.0085, -74.0182) (-151.0002, -74.9649) (-150.9916, -75.935) (-151.3508, -76.9039) (-151.9897, -77.634) knots -1 -1 -1 -1 -0.506107 -0.506107 -0.506107 0 0 0 0
  spline S4 degree 3 poles (-151.9897, -67.634) (-152.7286, -68.4785) (-153.8364, -68.9881) (-154.9584, -68.9998) (-156.1081, -69.0117) (-157.2531, -68.4994) (-158.0103, -67.634) knots -1 -1 -1 -1 -0.506107 -0.506107 -0.506107 0 0 0 0
  spline S5 degree 3 poles (-158.0103, -67.634) (-158.6337, -66.9215) (-158.9915, -65.9818) (-158.9998, -65.0351) (-159.0084, -64.065) (-158.6492, -63.0961) (-158.0103, -62.366) knots -1 -1 -1 -1 -0.506107 -0.506107 -0.506107 0 0 0 0
  spline S6 degree 3 poles (-158.0103, -62.366) (-157.2714, -61.5215) (-156.1636, -61.0119) (-155.0416, -61.0002) (-153.8919, -60.9883) (-152.7469, -61.5006) (-151.9897, -62.366) knots -1 -1 -1 -1 -0.506107 -0.506107 -0.506107 0 0 0 0
  spline S7 degree 3 poles (-151.9897, -62.366) (-151.3663, -63.0785) (-151.0085, -64.0182) (-151.0002, -64.9649) (-150.9916, -65.935) (-151.3508, -66.9039) (-151.9897, -67.634) knots -1 -1 -1 -1 -0.506107 -0.506107 -0.506107 0 0 0 0
  spline S8 degree 3 poles (-151.9897, -57.634) (-152.7286, -58.4785) (-153.8364, -58.9881) (-154.9584, -58.9998) (-156.1081, -59.0117) (-157.2531, -58.4994) (-158.0103, -57.634) knots -1 -1 -1 -1 -0.506107 -0.506107 -0.506107 0 0 0 0
  spline S9 degree 3 poles (-158.0103, -57.634) (-158.6337, -56.9215) (-158.9915, -55.9818) (-158.9998, -55.0351) (-159.0084, -54.065) (-158.6492, -53.0961) (-158.0103, -52.366) knots -1 -1 -1 -1 -0.506107 -0.506107 -0.506107 0 0 0 0
  spline S10 degree 3 poles (-158.0103, -52.366) (-157.2714, -51.5215) (-156.1636, -51.0119) (-155.0416, -51.0002) (-153.8919, -50.9883) (-152.7469, -51.5006) (-151.9897, -52.366) knots -1 -1 -1 -1 -0.506107 -0.506107 -0.506107 0 0 0 0
  spline S11 degree 3 poles (-151.9897, -52.366) (-151.3663, -53.0785) (-151.0085, -54.0182) (-151.0002, -54.9649) (-150.9916, -55.935) (-151.3508, -56.9039) (-151.9897, -57.634) knots -1 -1 -1 -1 -0.506107 -0.506107 -0.506107 0 0 0 0
  spline S12 degree 3 poles (-151.9897, -47.634) (-152.7286, -48.4785) (-153.8364, -48.9881) (-154.9584, -48.9998) (-156.1081, -49.0117) (-157.2531, -48.4994) (-158.0103, -47.634) knots -1 -1 -1 -1 -0.506107 -0.506107 -0.506107 0 0 0 0
  spline S13 degree 3 poles (-158.0103, -47.634) (-158.6337, -46.9215) (-158.9915, -45.9818) (-158.9998, -45.0351) (-159.0084, -44.065) (-158.6492, -43.0961) (-158.0103, -42.366) knots -1 -1 -1 -1 -0.506107 -0.506107 -0.506107 0 0 0 0
  spline S14 degree 3 poles (-158.0103, -42.366) (-157.2714, -41.5215) (-156.1636, -41.0119) (-155.0416, -41.0002) (-153.8919, -40.9883) (-152.7469, -41.5006) (-151.9897, -42.366) knots -1 -1 -1 -1 -0.506107 -0.506107 -0.506107 0 0 0 0
  spline S15 degree 3 poles (-151.9897, -42.366) (-151.3663, -43.0785) (-151.0085, -44.0182) (-151.0002, -44.9649) (-150.9916, -45.935) (-151.3508, -46.9039) (-151.9897, -47.634) knots -1 -1 -1 -1 -0.506107 -0.506107 -0.506107 0 0 0 0
  spline S16 degree 3 poles (-151.9897, -37.634) (-152.7286, -38.4785) (-153.8364, -38.9881) (-154.9584, -38.9998) (-156.1081, -39.0117) (-157.2531, -38.4994) (-158.0103, -37.634) knots -1 -1 -1 -1 -0.506107 -0.506107 -0.506107 0 0 0 0
  spline S17 degree 3 poles (-158.0103, -37.634) (-158.6337, -36.9215) (-158.9915, -35.9818) (-158.9998, -35.0351) (-159.0084, -34.065) (-158.6492, -33.0961) (-158.0103, -32.366) knots -1 -1 -1 -1 -0.506107 -0.506107 -0.506107 0 0 0 0
  spline S18 degree 3 poles (-158.0103, -32.366) (-157.2714, -31.5215) (-156.1636, -31.0119) (-155.0416, -31.0002) (-153.8919, -30.9883) (-152.7469, -31.5006) (-151.9897, -32.366) knots -1 -1 -1 -1 -0.506107 -0.506107 -0.506107 0 0 0 0
  spline S19 degree 3 poles (-151.9897, -32.366) (-151.3663, -33.0785) (-151.0085, -34.0182) (-151.0002, -34.9649) (-150.9916, -35.935) (-151.3508, -36.9039) (-151.9897, -37.634) knots -1 -1 -1 -1 -0.506107 -0.506107 -0.506107 0 0 0 0
  spline S20 degree 3 poles (-151.9897, -27.634) (-152.7286, -28.4785) (-153.8364, -28.9881) (-154.9584, -28.9998) (-156.1081, -29.0117) (-157.2531, -28.4994) (-158.0103, -27.634) knots -1 -1 -1 -1 -0.506107 -0.506107 -0.506107 0 0 0 0
  spline S21 degree 3 poles (-158.0103, -27.634) (-158.6337, -26.9215) (-158.9915, -25.9818) (-158.9998, -25.0351) (-159.0084, -24.065) (-158.6492, -23.0961) (-158.0103, -22.366) knots -1 -1 -1 -1 -0.506107 -0.506107 -0.506107 0 0 0 0
  spline S22 degree 3 poles (-158.0103, -22.366) (-157.2714, -21.5215) (-156.1636, -21.0119) (-155.0416, -21.0002) (-153.8919, -20.9883) (-152.7469, -21.5006) (-151.9897, -22.366) knots -1 -1 -1 -1 -0.506107 -0.506107 -0.506107 0 0 0 0
  spline S23 degree 3 poles (-151.9897, -22.366) (-151.3663, -23.0785) (-151.0085, -24.0182) (-151.0002, -24.9649) (-150.9916, -25.935) (-151.3508, -26.9039) (-151.9897, -27.634) knots -1 -1 -1 -1 -0.506107 -0.506107 -0.506107 0 0 0 0
  spline S24 degree 3 poles (-151.9897, -17.634) (-152.7286, -18.4785) (-153.8364, -18.9881) (-154.9584, -18.9998) (-156.1081, -19.0117) (-157.2531, -18.4994) (-158.0103, -17.634) knots -1 -1 -1 -1 -0.506107 -0.506107 -0.506107 0 0 0 0
  spline S25 degree 3 poles (-158.0103, -17.634) (-158.6337, -16.9215) (-158.9915, -15.9818) (-158.9998, -15.0351) (-159.0084, -14.065) (-158.6492, -13.0961) (-158.0103, -12.366) knots -1 -1 -1 -1 -0.506107 -0.506107 -0.506107 0 0 0 0
  spline S26 degree 3 poles (-158.0103, -12.366) (-157.2714, -11.5215) (-156.1636, -11.0119) (-155.0416, -11.0002) (-153.8919, -10.9883) (-152.7469, -11.5006) (-151.9897, -12.366) knots -1 -1 -1 -1 -0.506107 -0.506107 -0.506107 0 0 0 0
  spline S27 degree 3 poles (-151.9897, -12.366) (-151.3663, -13.0785) (-151.0085, -14.0182) (-151.0002, -14.9649) (-150.9916, -15.935) (-151.3508, -16.9039) (-151.9897, -17.634) knots -1 -1 -1 -1 -0.506107 -0.506107 -0.506107 0 0 0 0
  spline S28 degree 3 poles (-151.9897, -7.634) (-152.7286, -8.4785) (-153.8364, -8.9881) (-154.9584, -8.9998) (-156.1081, -9.0117) (-157.2531, -8.4994) (-158.0103, -7.634) knots -1 -1 -1 -1 -0.506107 -0.506107 -0.506107 0 0 0 0
  spline S29 degree 3 poles (-158.0103, -7.634) (-158.6337, -6.9215) (-158.9915, -5.9818) (-158.9998, -5.0351) (-159.0084, -4.065) (-158.6492, -3.0961) (-158.0103, -2.366) knots -1 -1 -1 -1 -0.506107 -0.506107 -0.506107 0 0 0 0
  spline S30 degree 3 poles (-158.0103, -2.366) (-157.2714, -1.5215) (-156.1636, -1.0119) (-155.0416, -1.0002) (-153.8919, -0.9883) (-152.7469, -1.5006) (-151.9897, -2.366) knots -1 -1 -1 -1 -0.506107 -0.506107 -0.506107 0 0 0 0
  spline S31 degree 3 poles (-151.9897, -2.366) (-151.3663, -3.0785) (-151.0085, -4.0182) (-151.0002, -4.9649) (-150.9916, -5.935) (-151.3508, -6.9039) (-151.9897, -7.634) knots -1 -1 -1 -1 -0.506107 -0.506107 -0.506107 0 0 0 0
  spline S32 degree 3 poles (-141.9897, -77.634) (-142.7286, -78.4785) (-143.8364, -78.9881) (-144.9584, -78.9998) (-146.1081, -79.0117) (-147.2531, -78.4994) (-148.0103, -77.634) knots -1 -1 -1 -1 -0.506107 -0.506107 -0.506107 0 0 0 0
  spline S33 degree 3 poles (-148.0103, -77.634) (-148.6337, -76.9215) (-148.9915, -75.9818) (-148.9998, -75.0351) (-149.0084, -74.065) (-148.6492, -73.0961) (-148.0103, -72.366) knots -1 -1 -1 -1 -0.506107 -0.506107 -0.506107 0 0 0 0
  spline S34 degree 3 poles (-148.0103, -72.366) (-147.2714, -71.5215) (-146.1636, -71.0119) (-145.0416, -71.0002) (-143.8919, -70.9883) (-142.7469, -71.5006) (-141.9897, -72.366) knots -1 -1 -1 -1 -0.506107 -0.506107 -0.506107 0 0 0 0
  spline S35 degree 3 poles (-141.9897, -72.366) (-141.3663, -73.0785) (-141.0085, -74.0182) (-141.0002, -74.9649) (-140.9916, -75.935) (-141.3508, -76.9039) (-141.9897, -77.634) knots -1 -1 -1 -1 -0.506107 -0.506107 -0.506107 0 0 0 0
  spline S36 degree 3 poles (-141.9897, -67.634) (-142.7286, -68.4785) (-143.8364, -68.9881) (-144.9584, -68.9998) (-146.1081, -69.0117) (-147.2531, -68.4994) (-148.0103, -67.634) knots -1 -1 -1 -1 -0.506107 -0.506107 -0.506107 0 0 0 0
  spline S37 degree 3 poles (-148.0103, -67.634) (-148.6337, -66.9215) (-148.9915, -65.9818) (-148.9998, -65.0351) (-149.0084, -64.065) (-148.6492, -63.0961) (-148.0103, -62.366) knots -1 -1 -1 -1 -0.506107 -0.506107 -0.506107 0 0 0 0
  spline S38 degree 3 poles (-148.0103, -62.366) (-147.2714, -61.5215) (-146.1636, -61.0119) (-145.0416, -61.0002) (-143.8919, -60.9883) (-142.7469, -61.5006) (-141.9897, -62.366) knots -1 -1 -1 -1 -0.506107 -0.506107 -0.506107 0 0 0 0
  spline S39 degree 3 poles (-141.9897, -62.366) (-141.3663, -63.0785) (-141.0085, -64.0182) (-141.0002, -64.9649) (-140.9916, -65.935) (-141.3508, -66.9039) (-141.9897, -67.634) knots -1 -1 -1 -1 -0.506107 -0.506107 -0.506107 0 0 0 0
  spline S40 degree 3 poles (-141.9897, -57.634) (-142.7286, -58.4785) (-143.8364, -58.9881) (-144.9584, -58.9998) (-146.1081, -59.0117) (-147.2531, -58.4994) (-148.0103, -57.634) knots -1 -1 -1 -1 -0.506107 -0.506107 -0.506107 0 0 0 0
  spline S41 degree 3 poles (-148.0103, -57.634) (-148.6337, -56.9215) (-148.9915, -55.9818) (-148.9998, -55.0351) (-149.0084, -54.065) (-148.6492, -53.0961) (-148.0103, -52.366) knots -1 -1 -1 -1 -0.506107 -0.506107 -0.506107 0 0 0 0
  spline S42 degree 3 poles (-148.0103, -52.366) (-147.2714, -51.5215) (-146.1636, -51.0119) (-145.0416, -51.0002) (-143.8919, -50.9883) (-142.7469, -51.5006) (-141.9897, -52.366) knots -1 -1 -1 -1 -0.506107 -0.506107 -0.506107 0 0 0 0
  spline S43 degree 3 poles (-141.9897, -52.366) (-141.3663, -53.0785) (-141.0085, -54.0182) (-141.0002, -54.9649) (-140.9916, -55.935) (-141.3508, -56.9039) (-141.9897, -57.634) knots -1 -1 -1 -1 -0.506107 -0.506107 -0.506107 0 0 0 0
  spline S44 degree 3 poles (-141.9897, -47.634) (-142.7286, -48.4785) (-143.8364, -48.9881) (-144.9584, -48.9998) (-146.1081, -49.0117) (-147.2531, -48.4994) (-148.0103, -47.634) knots -1 -1 -1 -1 -0.506107 -0.506107 -0.506107 0 0 0 0
  spline S45 degree 3 poles (-148.0103, -47.634) (-148.6337, -46.9215) (-148.9915, -45.9818) (-148.9998, -45.0351) (-149.0084, -44.065) (-148.6492, -43.0961) (-148.0103, -42.366) knots -1 -1 -1 -1 -0.506107 -0.506107 -0.506107 0 0 0 0
  spline S46 degree 3 poles (-148.0103, -42.366) (-147.2714, -41.5215) (-146.1636, -41.0119) (-145.0416, -41.0002) (-143.8919, -40.9883) (-142.7469, -41.5006) (-141.9897, -42.366) knots -1 -1 -1 -1 -0.506107 -0.506107 -0.506107 0 0 0 0
  spline S47 degree 3 poles (-141.9897, -42.366) (-141.3663, -43.0785) (-141.0085, -44.0182) (-141.0002, -44.9649) (-140.9916, -45.935) (-141.3508, -46.9039) (-141.9897, -47.634) knots -1 -1 -1 -1 -0.506107 -0.506107 -0.506107 0 0 0 0
  spline S48 degree 3 poles (-141.9897, -37.634) (-142.7286, -38.4785) (-143.8364, -38.9881) (-144.9584, -38.9998) (-146.1081, -39.0117) (-147.2531, -38.4994) (-148.0103, -37.634) knots -1 -1 -1 -1 -0.506107 -0.506107 -0.506107 0 0 0 0
  spline S49 degree 3 poles (-148.0103, -37.634) (-148.6337, -36.9215) (-148.9915, -35.9818) (-148.9998, -35.0351) (-149.0084, -34.065) (-148.6492, -33.0961) (-148.0103, -32.366) knots -1 -1 -1 -1 -0.506107 -0.506107 -0.506107 0 0 0 0
  spline S50 degree 3 poles (-148.0103, -32.366) (-147.2714, -31.5215) (-146.1636, -31.0119) (-145.0416, -31.0002) (-143.8919, -30.9883) (-142.7469, -31.5006) (-141.9897, -32.366) knots -1 -1 -1 -1 -0.506107 -0.506107 -0.506107 0 0 0 0
  spline S51 degree 3 poles (-141.9897, -32.366) (-141.3663, -33.0785) (-141.0085, -34.0182) (-141.0002, -34.9649) (-140.9916, -35.935) (-141.3508, -36.9039) (-141.9897, -37.634) knots -1 -1 -1 -1 -0.506107 -0.506107 -0.506107 0 0 0 0
  spline S52 degree 3 poles (-141.9897, -27.634) (-142.7286, -28.4785) (-143.8364, -28.9881) (-144.9584, -28.9998) (-146.1081, -29.0117) (-147.2531, -28.4994) (-148.0103, -27.634) knots -1 -1 -1 -1 -0.506107 -0.506107 -0.506107 0 0 0 0
  spline S53 degree 3 poles (-148.0103, -27.634) (-148.6337, -26.9215) (-148.9915, -25.9818) (-148.9998, -25.0351) (-149.0084, -24.065) (-148.6492, -23.0961) (-148.0103, -22.366) knots -1 -1 -1 -1 -0.506107 -0.506107 -0.506107 0 0 0 0
  spline S54 degree 3 poles (-148.0103, -22.366) (-147.2714, -21.5215) (-146.1636, -21.0119) (-145.0416, -21.0002) (-143.8919, -20.9883) (-142.7469, -21.5006) (-141.9897, -22.366) knots -1 -1 -1 -1 -0.506107 -0.506107 -0.506107 0 0 0 0
  spline S55 degree 3 poles (-141.9897, -22.366) (-141.3663, -23.0785) (-141.0085, -24.0182) (-141.0002, -24.9649) (-140.9916, -25.935) (-141.3508, -26.9039) (-141.9897, -27.634) knots -1 -1 -1 -1 -0.506107 -0.506107 -0.506107 0 0 0 0
  spline S56 degree 3 poles (-141.9897, -17.634) (-142.7286, -18.4785) (-143.8364, -18.9881) (-144.9584, -18.9998) (-146.1081, -19.0117) (-147.2531, -18.4994) (-148.0103, -17.634) knots -1 -1 -1 -1 -0.506107 -0.506107 -0.506107 0 0 0 0
  spline S57 degree 3 poles (-148.0103, -17.634) (-148.6337, -16.9215) (-148.9915, -15.9818) (-148.9998, -15.0351) (-149.0084, -14.065) (-148.6492, -13.0961) (-148.0103, -12.366) knots -1 -1 -1 -1 -0.506107 -0.506107 -0.506107 0 0 0 0
  spline S58 degree 3 poles (-148.0103, -12.366) (-147.2714, -11.5215) (-146.1636, -11.0119) (-145.0416, -11.0002) (-143.8919, -10.9883) (-142.7469, -11.5006) (-141.9897, -12.366) knots -1 -1 -1 -1 -0.506107 -0.506107 -0.506107 0 0 0 0
  spline S59 degree 3 poles (-141.9897, -12.366) (-141.3663, -13.0785) (-141.0085, -14.0182) (-141.0002, -14.9649) (-140.9916, -15.935) (-141.3508, -16.9039) (-141.9897, -17.634) knots -1 -1 -1 -1 -0.506107 -0.506107 -0.506107 0 0 0 0
  spline S60 degree 3 poles (-141.9897, -7.634) (-142.7286, -8.4785) (-143.8364, -8.9881) (-144.9584, -8.9998) (-146.1081, -9.0117) (-147.2531, -8.4994) (-148.0103, -7.634) knots -1 -1 -1 -1 -0.506107 -0.506107 -0.506107 0 0 0 0
  spline S61 degree 3 poles (-148.0103, -7.634) (-148.6337, -6.9215) (-148.9915, -5.9818) (-148.9998, -5.0351) (-149.0084, -4.065) (-148.6492, -3.0961) (-148.0103, -2.366) knots -1 -1 -1 -1 -0.506107 -0.506107 -0.506107 0 0 0 0
  spline S62 degree 3 poles (-148.0103, -2.366) (-147.2714, -1.5215) (-146.1636, -1.0119) (-145.0416, -1.0002) (-143.8919, -0.9883) (-142.7469, -1.5006) (-141.9897, -2.366) knots -1 -1 -1 -1 -0.506107 -0.506107 -0.506107 0 0 0 0
  spline S63 degree 3 poles (-141.9897, -2.366) (-141.3663, -3.0785) (-141.0085, -4.0182) (-141.0002, -4.9649) (-140.9916, -5.935) (-141.3508, -6.9039) (-141.9897, -7.634) knots -1 -1 -1 -1 -0.506107 -0.506107 -0.506107 0 0 0 0
  spline S64 degree 3 poles (-131.9897, -77.634) (-132.7286, -78.4785) (-133.8364, -78.9881) (-134.9584, -78.9998) (-136.1081, -79.0117) (-137.2531, -78.4994) (-138.0103, -77.634) knots -1 -1 -1 -1 -0.506107 -0.506107 -0.506107 0 0 0 0
  spline S65 degree 3 poles (-138.0103, -77.634) (-138.6337, -76.9215) (-138.9915, -75.9818) (-138.9998, -75.0351) (-139.0084, -74.065) (-138.6492, -73.0961) (-138.0103, -72.366) knots -1 -1 -1 -1 -0.506107 -0.506107 -0.506107 0 0 0 0
  spline S66 degree 3 poles (-138.0103, -72.366) (-137.2714, -71.5215) (-136.1636, -71.0119) (-135.0416, -71.0002) (-133.8919, -70.9883) (-132.7469, -71.5006) (-131.9897, -72.366) knots -1 -1 -1 -1 -0.506107 -0.506107 -0.506107 0 0 0 0
  spline S67 degree 3 poles (-131.9897, -72.366) (-131.3663, -73.0785) (-131.0085, -74.0182) (-131.0002, -74.9649) (-130.9916, -75.935) (-131.3508, -76.9039) (-131.9897, -77.634) knots -1 -1 -1 -1 -0.506107 -0.506107 -0.506107 0 0 0 0
  spline S68 degree 3 poles (-131.9897, -67.634) (-132.7286, -68.4785) (-133.8364, -68.9881) (-134.9584, -68.9998) (-136.1081, -69.0117) (-137.2531, -68.4994) (-138.0103, -67.634) knots -1 -1 -1 -1 -0.506107 -0.506107 -0.506107 0 0 0 0
  spline S69 degree 3 poles (-138.0103, -67.634) (-138.6337, -66.9215) (-138.9915, -65.9818) (-138.9998, -65.0351) (-139.0084, -64.065) (-138.6492, -63.0961) (-138.0103, -62.366) knots -1 -1 -1 -1 -0.506107 -0.506107 -0.506107 0 0 0 0
  spline S70 degree 3 poles (-138.0103, -62.366) (-137.2714, -61.5215) (-136.1636, -61.0119) (-135.0416, -61.0002) (-133.8919, -60.9883) (-132.7469, -61.5006) (-131.9897, -62.366) knots -1 -1 -1 -1 -0.506107 -0.506107 -0.506107 0 0 0 0
  spline S71 degree 3 poles (-131.9897, -62.366) (-131.3663, -63.0785) (-131.0085, -64.0182) (-131.0002, -64.9649) (-130.9916, -65.935) (-131.3508, -66.9039) (-131.9897, -67.634) knots -1 -1 -1 -1 -0.506107 -0.506107 -0.506107 0 0 0 0
  spline S72 degree 3 poles (-131.9897, -57.634) (-132.7286, -58.4785) (-133.8364, -58.9881) (-134.9584, -58.9998) (-136.1081, -59.0117) (-137.2531, -58.4994) (-138.0103, -57.634) knots -1 -1 -1 -1 -0.506107 -0.506107 -0.506107 0 0 0 0
  spline S73 degree 3 poles (-138.0103, -57.634) (-138.6337, -56.9215) (-138.9915, -55.9818) (-138.9998, -55.0351) (-139.0084, -54.065) (-138.6492, -53.0961) (-138.0103, -52.366) knots -1 -1 -1 -1 -0.506107 -0.506107 -0.506107 0 0 0 0
  spline S74 degree 3 poles (-138.0103, -52.366) (-137.2714, -51.5215) (-136.1636, -51.0119) (-135.0416, -51.0002) (-133.8919, -50.9883) (-132.7469, -51.5006) (-131.9897, -52.366) knots -1 -1 -1 -1 -0.506107 -0.506107 -0.506107 0 0 0 0
  spline S75 degree 3 poles (-131.9897, -52.366) (-131.3663, -53.0785) (-131.0085, -54.0182) (-131.0002, -54.9649) (-130.9916, -55.935) (-131.3508, -56.9039) (-131.9897, -57.634) knots -1 -1 -1 -1 -0.506107 -0.506107 -0.506107 0 0 0 0
  spline S76 degree 3 poles (-131.9897, -47.634) (-132.7286, -48.4785) (-133.8364, -48.9881) (-134.9584, -48.9998) (-136.1081, -49.0117) (-137.2531, -48.4994) (-138.0103, -47.634) knots -1 -1 -1 -1 -0.506107 -0.506107 -0.506107 0 0 0 0
  spline S77 degree 3 poles (-138.0103, -47.634) (-138.6337, -46.9215) (-138.9915, -45.9818) (-138.9998, -45.0351) (-139.0084, -44.065) (-138.6492, -43.0961) (-138.0103, -42.366) knots -1 -1 -1 -1 -0.506107 -0.506107 -0.506107 0 0 0 0
  spline S78 degree 3 poles (-138.0103, -42.366) (-137.2714, -41.5215) (-136.1636, -41.0119) (-135.0416, -41.0002) (-133.8919, -40.9883) (-132.7469, -41.5006) (-131.9897, -42.366) knots -1 -1 -1 -1 -0.506107 -0.506107 -0.506107 0 0 0 0